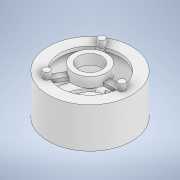
# Autodesk Inventor part: RobTrace_Wheel
Saved by Autodesk Inventor 2022 (Build 260153000, 153)
## iProperties
Created: 2021-09-21
Part Number: RobTrace_Wheel
Material: ABS プラスチック
Document SubType Name: Sheet Metal
Designer: youto
Density: 1.06 g/cm^3
Sheet Metal Rule: Default_mm
Appearance: 滑らか - 白
Author: youto
Autodesk Inventor part; units mm, degrees
ref_plane "YZ Plane" through (0, 0, 0) normal (1, 0, 0) x (0, 1, 0)
ref_plane "XZ Plane" through (0, 0, 0) normal (0, 1, 0) x (-1, 0, 0)
ref_plane "XY Plane" through (0, 0, 0) normal (0, 0, 1) x (1, 0, 0)
sketch "スケッチ1" plane through (0, 0, 0) normal (0, 1, 0) x (-1, 0, 0)
  circle A0 centre (-0.0357, -0.0516) radius 12.5
  circle A1 centre (-0.0357, -0.0516) radius 5
  circle A2 centre (-0.0357, -0.0516) radius 3.5
  circle A3 centre (-0.0357, -0.0516) radius 9
  arc A4 (-9.0357, -0.0516) -> (4.4643, -7.8458) centre (-0.0357, -0.0516) ccw
  line L0 (-0.0357, -0.0516) -> (4.4643, -7.8458) construction
  line L1 (-0.0357, -0.0516) -> (-9.0357, -0.0516) construction
  arc A5 (4.4643, 7.7426) -> (-9.0357, -0.0516) centre (-0.0357, -0.0516) ccw
  line L2 (-0.0357, -0.0516) -> (4.4643, 7.7426) construction
  line L3 (-0.0357, -0.0516) -> (-9.0357, -0.0516) construction
  line L4 (-9.0357, -0.0516) -> (-9.0357, 0.9484)
  line L5 (-9.0357, -0.0516) -> (-8.0357, -0.0516) construction
  line L6 (-9.0357, 0.9484) -> (-4.9347, 0.9484)
  line L7 (-9.0357, -0.0516) -> (-9.0357, -1.0516)
  line L8 (-9.0357, -0.0516) -> (-8.0357, -0.0516) construction
  line L9 (-9.0357, -1.0516) -> (-4.9347, -1.0516)
  line L10 (4.4643, 7.7426) -> (3.5983, 8.2426)
  line L11 (4.4643, 7.7426) -> (5.4643, 7.7426) construction
  line L12 (1.5477, 4.691) -> (3.5983, 8.2426)
  line L13 (4.4643, 7.7426) -> (5.3012, 7.1953)
  line L14 (5.3012, 7.1953) -> (3.2798, 3.691)
  line L15 (4.4643, -7.8458) -> (3.5983, -8.3458)
  line L16 (4.4643, -7.8458) -> (5.4643, -7.8458) construction
  line L17 (3.5983, -8.3458) -> (1.5477, -4.7942)
  line L18 (4.4643, -7.8458) -> (5.3303, -7.3458)
  line L19 (4.4643, -7.8458) -> (5.4643, -7.8458) construction
  line L20 (5.3303, -7.3458) -> (3.2798, -3.7942)
  circle A6 centre (-0.0357, -0.0516) radius 12
  point P0 (0, 0)
  point P1 (-9.0357, -0.0516)
  point P2 (3.5704, -8.2976)
  point P3 (-8.98, -1.0516)
  point P4 (-8.98, 0.9484)
  point P5 (3.5704, 8.1944)
  point P6 (5.3024, -7.2976)
  dimension "d1" = 25
  dimension "d2" = 10
  dimension "d3" = 7
  dimension "d4" = 18
  dimension "d5" = 120
  dimension "d6" = 120
  dimension "d7" = 1
  dimension "d8" = 90
  dimension "d9" = 1
  dimension "d10" = 90
  dimension "d11" = 1
  dimension "d12" = 150
  dimension "d13" = 1
  dimension "d14" = 1
  dimension "d15" = 150
  dimension "d16" = 1
  dimension "d17" = 30
  dimension "d18" = 24
  constraints: 42 end point, 13 point on circle, 11 coincident, 8 tangent, 7 centre point, 7 horizontal, 5 equal length, 2 perpendicular, 1 parallel
  measures "d1" diameter of A0
  measures "d2" diameter of A1
  measures "d3" diameter of A2
  measures "d4" diameter of A3
  measures "d5" angle of L1 L0
  measures "d6" angle of L2 L3
  measures "d7" distance of L1.end L4.end
  measures "d8" angle of L5 L4
  measures "d9" distance of L1.end L7.end
  measures "d10" angle of L7 L8
  measures "d11" distance of L2.end L10.end
  measures "d12" angle of L11 L10
  measures "d13" distance of L2.end L13.end
  measures "d14" distance of L0.end L15.end
  measures "d15" angle of L15 L16
  measures "d16" distance of L0.end L18.end
  measures "d17" angle of L19 L18
  measures "d18" diameter of A6
extrude "押し出し1" add sketch "スケッチ1" along normal blind 12 contours A0
extrude "押し出し2" add sketch "スケッチ1" along normal blind 1 contours A1 L12 A3 L13 L14 | L20 A3 L17 A1 | L13 A3 | L20 L18 A3 | A1 L9 A3 L6 | L12 L10 A3 | A3 L15 L17 | A3 L4 L6 | L9 L7 A3 | A6
extrude "押し出し3" add sketch "スケッチ1" along normal blind 3 contours A1
extrude "押し出し4" add sketch "スケッチ1" against normal blind 1 from surface at 12 contours A1 | A1 L12 A3 L13 L14 | L20 A3 L17 A1 | L13 A3 | L20 L18 A3 | A1 L9 A3 L6 | L12 L10 A3 | A3 L15 L17 | A3 L4 L6 | L9 L7 A3 | A6
extrude "押し出し5" add sketch "スケッチ1" along normal blind 2 from surface at 12 contours A1
sketch "スケッチ2" plane through (0.0357, 12, -0.0516) normal (0, 1, 0) x (1, 0, 0)
  circle A0 centre (0, 0) radius 9.5
  arc A1 (-4.75, -8.2272) -> (9.5, 0) centre (0, 0) ccw
  line L0 (0, 0) -> (-4.75, -8.2272) construction
  line L1 (0, 0) -> (9.5, 0) construction
  arc A2 (9.5, 0) -> (-4.75, 8.2272) centre (0, 0) ccw
  line L2 (0, 0) -> (-4.75, 8.2272) construction
  line L3 (0, 0) -> (9.5, 0) construction
  circle A3 centre (9.5, 0) radius 1
  circle A4 centre (-4.75, -8.2272) radius 1
  circle A5 centre (-4.75, 8.2272) radius 1
  point P0 (-0.0357, -0.0516)
  dimension "d29" = 19
  dimension "d30" = 120
  dimension "d31" = 120
  dimension "d32" = 2
  dimension "d33" = 2
  dimension "d34" = 2
  constraints: 8 end point, 5 centre point, 5 coincident, 4 point on circle, 1 horizontal alignment, 2 other
  measures "d30" angle of L0 L1
  measures "d31" angle of L3 L2
  measures "d32" diameter of A3
  measures "d33" diameter of A4
  measures "d34" diameter of A5
extrude "押し出し6" add sketch "スケッチ2" along normal blind 2 contours A0 A3 | A0 A3 | A5 A0 | A0 A5 | A4 A0 | A0 A4
equation "\"BendRadius\" = Thickness"
equation "\"BendReliefWidth\" = Thickness"
equation "\"BendReliefDepth\" = 0.5 * Thickness"
equation "\"CornerReliefSize\" = 4 * Thickness"
equation "\"MinimumRemnant\" = 2 * Thickness"
equation "\"TransitionRadius\" = BendRadius"
equation "\"JacobiRadiusSize\" = BendRadius"
equation "\"GapSize\" = Thickness"
equation "\"Thickness\" = 0.5"
